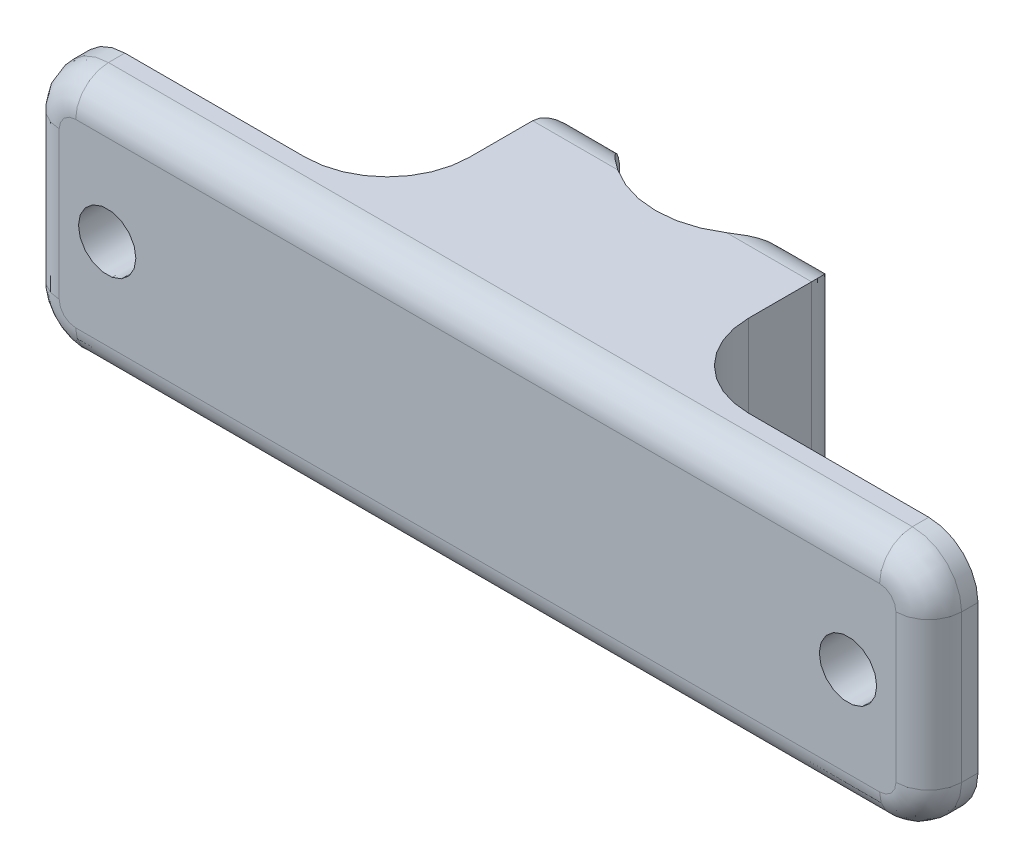
# Autodesk Inventor part: PlotterPenHolderAltClamp
Saved by Autodesk Inventor 2018 (Build 220112000, 112)
## iProperties
Created: 2018-05-11
Part Number: PlotterPenHolderAltClamp
Material: Generic
Document SubType Name: Modeling
Designer: Jasper
Density: 1 g/cm^3
Appearance: Default
Author: Jasper
Autodesk Inventor part; units mm, degrees
ref_plane "YZ Plane" through (0, 0, 0) normal (1, 0, 0) x (0, 1, 0)
ref_plane "XZ Plane" through (0, 0, 0) normal (0, 1, 0) x (-1, 0, 0)
ref_plane "XY Plane" through (0, 0, 0) normal (0, 0, 1) x (1, 0, 0)
sketch "Sketch1" plane through (0, 0, 0) normal (0, 0, 1) x (1, 0, 0)
  point P0 (0, 0)
sketch "Sketch2" plane through (0, 0, 0) normal (0, 0, 1) x (1, 0, 0)
  line L0 (-27.5, 7.5) -> (27.5, 7.5)
  line L1 (27.5, 7.5) -> (27.5, -7.5)
  line L2 (27.5, -7.5) -> (-27.5, -7.5)
  line L3 (-27.5, -7.5) -> (-27.5, 7.5)
  line L4 (-27.5, 7.5) -> (27.5, -7.5) construction
  line L5 (27.5, 7.5) -> (-27.5, -7.5) construction
  point P0 (0, 0)
  dimension "d0" = 15
  dimension "d1" = 55
  constraints: 12 end point, 2 midpoint, 2 parallel, 1 horizontal, 1 perpendicular
  measures "d0" distance of L2.end L0.start
  measures "d1" distance of L0.start L0.end
extrude "Extrusion1" add sketch "Sketch2" along normal blind 3
sketch "Sketch3" plane through (0, 0, 3) normal (0, 0, 1) x (1, 0, 0)
  line L0 (0, 0) -> (22.5765, 0) construction
  circle A0 centre (22.5765, 0) radius 1.75
  line L1 (27.5, 7.5) -> (-27.5, 7.5) construction
  line L2 (0, 7.5) -> (0, -7.5) construction
  line L3 (-27.5, -7.5) -> (27.5, -7.5) construction
  line L4 (0, 0) -> (-22.5765, 0) construction
  circle A1 centre (-22.5765, 0) radius 1.75
  dimension "d4" = 3.5
  dimension "d5" = 45.153
  constraints: 6 end point, 2 centre point, 2 coincident, 2 midpoint, 2 symmetric about line, 1 horizontal, 1 other
  measures "d4" diameter of A0
  measures "d5" distance of L4.end L0.end
extrude "Extrusion2" cut sketch "Sketch3" against normal through all
sketch "Sketch4" plane through (-27.5, 7.5, 0) normal (0, 1, 0) x (1, 0, 0)
  line L0 (55, 0) -> (0, 0) projected
  line L1 (19, 0) -> (19, 10.8562)
  line L2 (36, 0) -> (36, 10.8562)
  line L3 (27.5, 10.8562) -> (27.5, 0) construction
  line L4 (19, 7.8562) -> (36, 7.8562) construction
  line L5 (19, 0) -> (36, 0) construction
  line L6 (19, 0) -> (36, 0)
  line L7 (19, 10.8562) -> (36, 10.8562) construction
  circle A0 centre (27.5, 13.8562) radius 6
  line L8 (19, 10.8562) -> (22.3038, 10.8562)
  line L9 (36, 10.8562) -> (32.6962, 10.8562)
  dimension "d10" = 10.8562
  dimension "d11" = 17
  dimension "d12" = 12
  dimension "d13" = 3
  constraints: 18 end point, 7 point on line, 3 perpendicular, 2 collinear, 2 point on circle, 1 centre point, 1 parallel, 1 tangent, 1 vertical, 1 other
  measures "d10" distance of L1.start L1.end
  measures "d11" distance between parallel lines of L1 L2
  measures "d12" diameter of A0
  measures "d13" distance between parallel lines of L7 L4
extrude "Extrusion3" add sketch "Sketch4" against normal up to surface (15 mm away) contours L0 L1 L8 A0 L9 L2
fillet "Fillet1" radius 3 4 edges at (-27.5, 7.5, 1.5) (-27.5, -7.5, 1.5) (27.5, 7.5, 1.5) (27.5, -7.5, 1.5)
fillet "Fillet2" radius 2 8 edges at (-26.6213, 6.6213, 3) (-27.5, 0, 3) (-26.6213, -6.6213, 3) (0, -7.5, 3) (26.6213, -6.6213, 3) (27.5, 0, 3) (26.6213, 6.6213, 3) (0, 7.5, 3)
fillet "Fillet3" radius 5 2 edges at (-8.5, 0, 0) (8.5, 0, 0)
fillet "Fillet4" radius 2 6 edges at (-6.8481, 7.5, -10.8562) (-8.5, 0, -10.8562) (8.5, 0, -10.8562) (-6.8481, -7.5, -10.8562) (6.8481, -7.5, -10.8562) (6.8481, 7.5, -10.8562)
body "Solid1"
